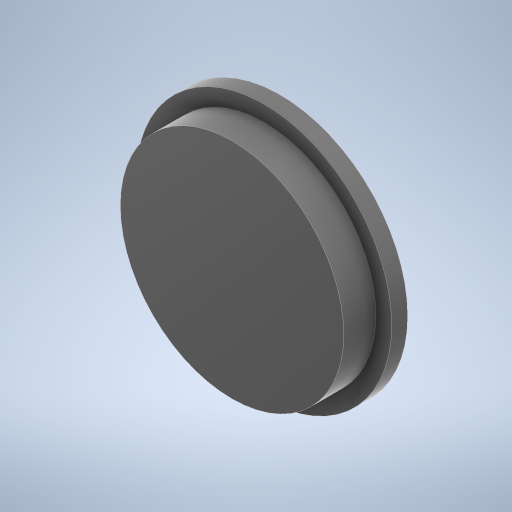
# Autodesk Inventor part: pokrywka
Saved by Autodesk Inventor 2024 (Build 280153000, 153)
## iProperties
Created: 2025-05-20
Part Number: pokrywka
Material: Tworzywo sztuczne PET
Document SubType Name: Modeling
Designer: Paweł
Density: 1.541 g/cm^3
Appearance: Gładki — czarny
Mass: 98.0342 g
Surface Area: 135.088 cm^2
Volume: 63.6173 cm^3
Author: Paweł
Autodesk Inventor part; units mm, degrees
ref_plane "YZ Plane" through (0, 0, 0) normal (1, 0, 0) x (0, 1, 0)
ref_plane "XZ Plane" through (0, 0, 0) normal (0, 1, 0) x (-1, 0, 0)
ref_plane "XY Plane" through (0, 0, 0) normal (0, 0, 1) x (1, 0, 0)
sketch "Szkic1" plane through (0, 0, 0) normal (0, 0, 1) x (1, 0, 0)
  circle A0 centre (0, 0) radius 40
  circle A1 centre (0, 0) radius 35
  dimension "d0" = 80
  dimension "d1" = 5
  constraints: 2 centre point, 1 coincident
  measures "d0" diameter of A0
  measures "d1" radial gap between concentric circles of A0 A1
extrude "Wyciągnięcie proste1" add sketch "Szkic1" along normal blind 5 contours A0 | A1
sketch "Szkic2" plane through (0, 0, 5) normal (0, 0, 1) x (1, 0, 0)
  circle A0 centre (0, 0) radius 40 projected
  circle A1 centre (0, 0) radius 35
  dimension "d4" = 5
  constraints: 1 centre point
  measures "d4" radial gap between concentric circles of A0 A1
extrude "Wyciągnięcie proste2" add sketch "Szkic2" along normal blind 10 contours A1
